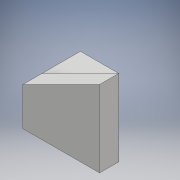
# Autodesk Inventor part: 3
Saved by Autodesk Inventor 2017 (Build 210142000, 142)
## iProperties
Part Number: 3
Material: 一般
Document SubType Name: Modeling
Designer: Brian
Density: 1 g/cm^3
Appearance: 預設
Author: Brian
Autodesk Inventor part; units mm, degrees
ref_plane "YZ Plane" through (0, 0, 0) normal (1, 0, 0) x (0, 1, 0)
ref_plane "XZ Plane" through (0, 0, 0) normal (0, 1, 0) x (-1, 0, 0)
ref_plane "XY Plane" through (0, 0, 0) normal (0, 0, 1) x (1, 0, 0)
sketch "草圖1" plane through (0, 0, 0) normal (0, 1, 0) x (-1, 0, 0)
  line L0 (0, 0) -> (0, -20)
  line L1 (0, -20) -> (-40, -20)
  line L2 (-40, -20) -> (-40, 20)
  line L3 (-40, 20) -> (0, 0)
  dimension "d0" = 40
  dimension "d1" = 20
  dimension "d2" = 40
  constraints: 8 end point, 2 vertical, 1 perpendicular
  measures "d0" distance of L1.end L2.end
  measures "d1" distance of L0.start L0.end
  measures "d2" distance of L0.end L1.end
extrude "擠出1" add sketch "草圖1" along normal blind 10
sketch "草圖2" plane through (0, 10, 0) normal (0, 1, 0) x (1, 0, 0)
  line L0 (0, 0) -> (20, 0)
  line L1 (20, 0) -> (20, 20)
  line L2 (20, 20) -> (0, 20)
  line L3 (0, 20) -> (0, 0)
  dimension "d5" = 20
  dimension "d6" = 20
  constraints: 8 end point, 2 parallel, 1 horizontal, 1 perpendicular
  measures "d5" distance of L0.end L1.end
  measures "d6" distance of L0.start L0.end
extrude "擠出2" add sketch "草圖2" along normal blind 20
